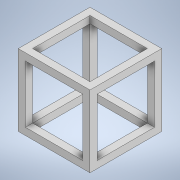
# Autodesk Inventor part: Cube
Saved by Autodesk Inventor 2022 (Build 260153000, 153)
## iProperties
Created: 2022-02-15
Part Number: Cube
Material: Generic
Document SubType Name: Modeling
Designer: Nathan Griffith
Density: 1 g/cm^3
Appearance: Default
Author: Nathan Griffith
Autodesk Inventor part; units mm, degrees
ref_plane "YZ Plane" through (0, 0, 0) normal (1, 0, 0) x (0, 1, 0)
ref_plane "XZ Plane" through (0, 0, 0) normal (0, 1, 0) x (-1, 0, 0)
ref_plane "XY Plane" through (0, 0, 0) normal (0, 0, 1) x (1, 0, 0)
sketch "Sketch1" plane through (0, 0, 0) normal (0, 1, 0) x (-1, 0, 0)
  line L0 (-31.75, -31.75) -> (31.75, -31.75)
  line L1 (31.75, -31.75) -> (31.75, 31.75)
  line L2 (31.75, 31.75) -> (-31.75, 31.75)
  line L3 (-31.75, 31.75) -> (-31.75, -31.75)
  line L4 (-31.75, -31.75) -> (31.75, 31.75) construction
  line L5 (31.75, -31.75) -> (-31.75, 31.75) construction
  point P0 (0, 0)
  dimension "d0" = 63.5
  dimension "d1" = 63.5
  constraints: 12 end point, 2 midpoint, 2 parallel, 1 horizontal, 1 perpendicular
  measures "d0" distance of L2.end L1.end
  measures "d1" distance of L1.end L0.end
extrude "Extrusion1" add sketch "Sketch1" along normal blind 63.5
sketch "Sketch2" plane through (31.75, 0, 31.75) normal (1, 0, 0) x (0, 0, -1)
  line L0 (63.5, 63.5) -> (0, 63.5) projected
  line L1 (31.75, 63.5) -> (31.75, 0)
  line L2 (0, 0) -> (0, 63.5) projected
  line L3 (0, 31.75) -> (63.5, 31.75)
  line L4 (0, 0) -> (0, 63.5) projected
  line L5 (63.5, 0) -> (63.5, 63.5) projected
  line L6 (57.15, 6.35) -> (6.35, 6.35)
  line L7 (6.35, 6.35) -> (6.35, 57.15)
  line L8 (6.35, 57.15) -> (57.15, 57.15)
  line L9 (57.15, 57.15) -> (57.15, 6.35)
  line L10 (57.15, 6.35) -> (6.35, 57.15) construction
  line L11 (6.35, 6.35) -> (57.15, 57.15) construction
  line L12 (0, 63.5) -> (63.5, 63.5) projected
  line L13 (0, 0) -> (63.5, 0) projected
  point P0 (0, 31.75)
  point P1 (63.5, 31.75)
  point P2 (31.75, 31.75)
  point P3 (31.75, 63.5)
  dimension "d4" = 50.8
  dimension "d5" = 50.8
  constraints: 16 end point, 10 midpoint, 2 horizontal, 2 parallel, 1 perpendicular, 1 point on line, 1 vertical
  measures "d4" distance of L7.end L8.end
  measures "d5" distance of L6.end L7.end
extrude "Extrusion2" cut sketch "Sketch2" against normal through all contours L8 L9 L3 L1 | L1 L3 L7 L8 | L9 L6 L1 L3 | L1 L6 L7 L3
sketch "Sketch3" plane through (0, 63.5, 0) normal (0, 1, 0) x (1, 0, 0)
  line L0 (25.4, -25.4) -> (-25.4, -25.4)
  line L1 (-25.4, -25.4) -> (-25.4, 25.4)
  line L2 (-25.4, 25.4) -> (25.4, 25.4)
  line L3 (25.4, 25.4) -> (25.4, -25.4)
  line L4 (25.4, -25.4) -> (-25.4, 25.4) construction
  line L5 (-25.4, -25.4) -> (25.4, 25.4) construction
  point P0 (0, 0)
  dimension "d8" = 50.8
  dimension "d9" = 50.8
  constraints: 12 end point, 2 midpoint, 2 parallel, 1 horizontal, 1 perpendicular
  measures "d8" distance of L1.end L2.end
  measures "d9" distance of L0.end L1.end
extrude "Extrusion3" cut sketch "Sketch3" against normal through all
sketch "Sketch4" plane through (31.75, 0, -31.75) normal (0, 0, -1) x (-1, 0, 0)
  line L0 (63.5, 6.35) -> (63.5, 57.15) projected
  line L1 (63.5, 31.75) -> (0, 31.75)
  line L2 (0, 0) -> (0, 63.5) projected
  line L3 (6.35, 63.5) -> (57.15, 63.5) projected
  line L4 (31.75, 63.5) -> (31.75, 0)
  line L5 (6.35, 6.35) -> (57.15, 6.35)
  line L6 (57.15, 6.35) -> (57.15, 57.15)
  line L7 (57.15, 57.15) -> (6.35, 57.15)
  line L8 (6.35, 57.15) -> (6.35, 6.35)
  line L9 (6.35, 6.35) -> (57.15, 57.15) construction
  line L10 (57.15, 6.35) -> (6.35, 57.15) construction
  point P0 (31.75, 31.75)
  dimension "d12" = 50.8
  dimension "d13" = 50.8
  constraints: 16 end point, 6 midpoint, 2 parallel, 1 horizontal, 1 perpendicular, 1 vertical
  measures "d12" distance of L7.end L6.end
  measures "d13" distance of L6.end L5.end
extrude "Extrusion4" cut sketch "Sketch4" against normal through all
body "Solid1"
